Autodesk Inventor part; units mm, degrees
(part 3 of 3)
  constraints: 48 tangent, 16 centre point
hole "Hole1" at (-1360.7789, 0.6205, -2600.6334) at (-1305.7789, 0.6205, -2600.6334) at (-1235.7789, 0.6204, -2600.6334) at (-1235.7789, -54.3796, -2600.6334) at (-1305.7789, -54.3795, -2600.6334) at (-1305.7789, -185.4295, -2600.6334) at (-1235.7789, -185.4295, -2600.6334) at (-1235.7789, -314.3795, -2600.6334) at (-1305.7789, -314.3795, -2600.6334) at (-1305.7789, -443.3295, -2600.6334) at (-1235.7789, -443.3296, -2600.6334) at (-1235.7789, -574.3795, -2600.6334) at (-1305.7789, -574.3795, -2600.6334) at (-1360.7789, -629.3795, -2600.6334) at (-1305.7789, -629.3795, -2600.6334) at (-1235.7789, -629.3795, -2600.6334) direction (0, 0, 1) diameter 5.2 end through all
body "Solid1"
